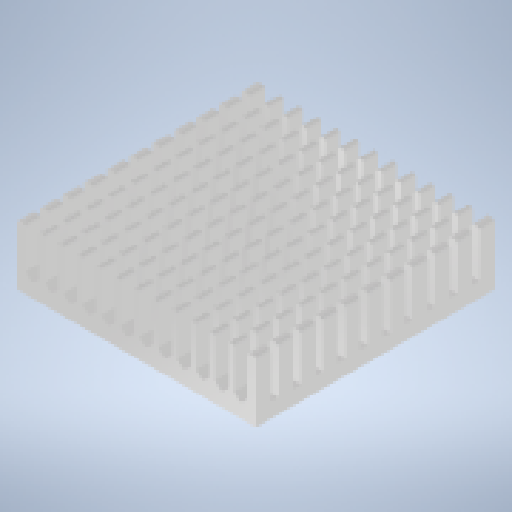
# Autodesk Inventor part: Nema17_CoolingElement
Saved by Autodesk Inventor 2023.1 (Build 271208000, 208)
## iProperties
Created: 2022-09-11
Part Number: Nema17_CoolingElement
Material: Generisch
Document SubType Name: Modeling
Designer: Rama
Density: 1 g/cm^3
Appearance: Aluminium - dunkel
Author: Rama
Autodesk Inventor part; units mm, degrees
ref_plane "YZ Plane" through (0, 0, 0) normal (1, 0, 0) x (0, 1, 0)
ref_plane "XZ Plane" through (0, 0, 0) normal (0, 1, 0) x (-1, 0, 0)
ref_plane "XY Plane" through (0, 0, 0) normal (0, 0, 1) x (1, 0, 0)
sketch "Skizze1" plane through (0, 0, 0) normal (0, 0, 1) x (1, 0, 0)
  line L0 (0, 4.4) -> (2, 4.4) projected
  line L1 (0, 0.4) -> (0, 4.4) projected
  line L2 (40.4, 0.4) -> (0, 0.4) projected
  line L3 (40.4, 0.4) -> (40.4, 4.4) projected
  line L4 (38.4, 4.4) -> (40.4, 4.4) projected
  line L5 (38.4, 3) -> (38.4, 4.4) projected
  line L6 (38, 2.6) -> (38.4, 3) projected
  line L7 (37.6, 2.6) -> (38, 2.6) projected
  line L8 (37.2, 3) -> (37.6, 2.6) projected
  line L9 (37.2, 3) -> (37.2, 4.4) projected
  line L10 (35.2, 4.4) -> (37.2, 4.4) projected
  line L11 (35.2, 3) -> (35.2, 4.4) projected
  line L12 (34.8, 2.6) -> (35.2, 3) projected
  line L13 (34.4, 2.6) -> (34.8, 2.6) projected
  line L14 (34, 3) -> (34.4, 2.6) projected
  line L15 (34, 3) -> (34, 4.4) projected
  line L16 (32, 4.4) -> (34, 4.4) projected
  line L17 (32, 3) -> (32, 4.4) projected
  line L18 (31.6, 2.6) -> (32, 3) projected
  line L19 (31.2, 2.6) -> (31.6, 2.6) projected
  line L20 (30.8, 3) -> (31.2, 2.6) projected
  line L21 (30.8, 3) -> (30.8, 4.4) projected
  line L22 (28.8, 4.4) -> (30.8, 4.4) projected
  line L23 (28.8, 3) -> (28.8, 4.4) projected
  line L24 (28.4, 2.6) -> (28.8, 3) projected
  line L25 (28, 2.6) -> (28.4, 2.6) projected
  line L26 (27.6, 3) -> (28, 2.6) projected
  line L27 (27.6, 3) -> (27.6, 4.4) projected
  line L28 (25.6, 4.4) -> (27.6, 4.4) projected
  line L29 (25.6, 3) -> (25.6, 4.4) projected
  line L30 (25.2, 2.6) -> (25.6, 3) projected
  line L31 (24.8, 2.6) -> (25.2, 2.6) projected
  line L32 (24.4, 3) -> (24.8, 2.6) projected
  line L33 (24.4, 3) -> (24.4, 4.4) projected
  line L34 (22.4, 4.4) -> (24.4, 4.4) projected
  line L35 (22.4, 3) -> (22.4, 4.4) projected
  line L36 (22, 2.6) -> (22.4, 3) projected
  line L37 (21.6, 2.6) -> (22, 2.6) projected
  line L38 (21.2, 3) -> (21.6, 2.6) projected
  line L39 (21.2, 3) -> (21.2, 4.4) projected
  line L40 (19.2, 4.4) -> (21.2, 4.4) projected
  line L41 (19.2, 3) -> (19.2, 4.4) projected
  line L42 (18.8, 2.6) -> (19.2, 3) projected
  line L43 (18.4, 2.6) -> (18.8, 2.6) projected
  line L44 (18, 3) -> (18.4, 2.6) projected
  line L45 (18, 3) -> (18, 4.4) projected
  line L46 (16, 4.4) -> (18, 4.4) projected
  line L47 (16, 3) -> (16, 4.4) projected
  line L48 (15.6, 2.6) -> (16, 3) projected
  line L49 (15.2, 2.6) -> (15.6, 2.6) projected
  line L50 (14.8, 3) -> (15.2, 2.6) projected
  line L51 (14.8, 3) -> (14.8, 4.4) projected
  line L52 (12.8, 4.4) -> (14.8, 4.4) projected
  line L53 (12.8, 3) -> (12.8, 4.4) projected
  line L54 (12.4, 2.6) -> (12.8, 3) projected
  line L55 (12, 2.6) -> (12.4, 2.6) projected
  line L56 (11.6, 3) -> (12, 2.6) projected
  line L57 (11.6, 3) -> (11.6, 4.4) projected
  line L58 (9.6, 4.4) -> (11.6, 4.4) projected
  line L59 (9.6, 3) -> (9.6, 4.4) projected
  line L60 (9.2, 2.6) -> (9.6, 3) projected
  line L61 (8.8, 2.6) -> (9.2, 2.6) projected
  line L62 (8.4, 3) -> (8.8, 2.6) projected
  line L63 (8.4, 3) -> (8.4, 4.4) projected
  line L64 (6.4, 4.4) -> (8.4, 4.4) projected
  line L65 (6.4, 3) -> (6.4, 4.4) projected
  line L66 (6, 2.6) -> (6.4, 3) projected
  line L67 (5.6, 2.6) -> (6, 2.6) projected
  line L68 (5.2, 3) -> (5.6, 2.6) projected
  line L69 (5.2, 3) -> (5.2, 4.4) projected
  line L70 (3.2, 4.4) -> (5.2, 4.4) projected
  line L71 (3.2, 3) -> (3.2, 4.4) projected
  line L72 (2.8, 2.6) -> (3.2, 3) projected
  line L73 (2.4, 2.6) -> (2.8, 2.6) projected
  line L74 (2, 3) -> (2.4, 2.6) projected
  line L75 (2, 3) -> (2, 4.4) projected
  line L76 (40.4, 0.4) -> (0, 0.4)
  line L77 (0, 0.4) -> (0, -0.4)
  line L78 (0, -0.4) -> (40.4, -0.4)
  line L79 (40.4, -0.4) -> (40.4, 0.4)
  point P0 (0, 0)
  dimension "d0" = 0.8
  constraints: 8 end point, 2 parallel, 1 horizontal, 1 perpendicular, 1 point on line
  measures "d0" distance between parallel lines of L76 L78
ref_plane "Arbeitsebene1" through (0, 0.4, 40.4) normal (0, 0, -1) x (0, 1, 0)
extrude "Extrusion1" add sketch "Skizze1" along normal up to surface (40.4 mm away)
chamfer "Fase1" distance 0.5 angle 45 4 edges at (0, -0.4, 20.2) (20.2, -0.4, 0) (40.4, -0.4, 20.2) (20.2, -0.4, 40.4)
move faces "Verschieben1" translate (0, 6, 0) faces at (1.3333, 4.4, 13.4667) (4.5333, 4.4, 13.4667) (7.7333, 4.4, 13.4667) (10.9333, 4.4, 13.4667) (14.1333, 4.4, 13.4667) (17.3333, 4.4, 13.4667) (20.5333, 4.4, 13.4667) (23.7333, 4.4, 13.4667) (26.9333, 4.4, 13.4667) (30.1333, 4.4, 13.4667) (33.3333, 4.4, 13.4667) (36.5333, 4.4, 13.4667) (39.7333, 4.4, 13.4667)
move faces "Verschieben2" translate (-0.5, 0, 0) faces at (37.2, 5.4667, 13.4667) (34, 5.4667, 13.4667) (30.8, 5.4667, 13.4667) (27.6, 5.4667, 13.4667) (24.4, 5.4667, 13.4667) (21.2, 5.4667, 13.4667) (18, 5.4667, 13.4667) (14.8, 5.4667, 13.4667) (11.6, 5.4667, 13.4667) (8.4, 5.4667, 13.4667) (5.2, 5.4667, 13.4667) (2, 5.4667, 13.4667)
move faces "Verschieben3" translate (0.5, 0, 0) faces at (3.2, 7.9333, 13.4667) (6.4, 7.9333, 13.4667) (9.6, 7.9333, 13.4667) (12.8, 5.4667, 26.9333) (16, 7.9333, 13.4667) (19.2, 5.4667, 26.9333) (22.4, 5.4667, 26.9333) (25.6, 7.9333, 13.4667) (28.8, 7.9333, 13.4667) (32, 7.9333, 13.4667) (35.2, 7.9333, 13.4667) (38.4, 7.9333, 13.4667)
fillet "Rundung1" radius 0.5 26 edges at (0, 10.4, 20.2) (1.5, 10.4, 20.2) (3.7, 10.4, 20.2) (4.7, 10.4, 20.2) (6.9, 10.4, 20.2) (7.9, 10.4, 20.2) (10.1, 10.4, 20.2) (11.1, 10.4, 20.2) (13.3, 10.4, 20.2) (14.3, 10.4, 20.2) (16.5, 10.4, 20.2) (17.5, 10.4, 20.2) (19.7, 10.4, 20.2) (20.7, 10.4, 20.2) (22.9, 10.4, 20.2) (23.9, 10.4, 20.2) (26.1, 10.4, 20.2) (27.1, 10.4, 20.2) (29.3, 10.4, 20.2) (30.3, 10.4, 20.2) (32.5, 10.4, 20.2) (33.5, 10.4, 20.2) (35.7, 10.4, 20.2) (36.7, 10.4, 20.2) (38.9, 10.4, 20.2) (40.4, 10.4, 20.2)
sketch "Skizze2" plane through (0, 0.1, 0) normal (-1, 0, 0) x (0, 0, 1)
  line L0 (0, 9.8) -> (40.4, 9.8) projected
  line L1 (0, 9.8) -> (0, 0) projected
  line L2 (40.4, 0) -> (0, 0) projected
  line L3 (40.4, 9.8) -> (40.4, 0) projected
  line L4 (37.9, 2.5) -> (36.61, 2.5)
  line L5 (36.61, 2.5) -> (36.61, 12.7645)
  line L6 (36.61, 12.7645) -> (37.9, 12.7645)
  line L7 (37.9, 12.7645) -> (37.9, 2.5)
  line L8 (34.11, 2.5) -> (32.82, 2.5)
  line L9 (32.82, 2.5) -> (32.82, 12.7645)
  line L10 (32.82, 12.7645) -> (34.11, 12.7645)
  line L11 (34.11, 12.7645) -> (34.11, 2.5)
  line L12 (30.32, 2.5) -> (29.03, 2.5)
  line L13 (29.03, 2.5) -> (29.03, 12.7645)
  line L14 (29.03, 12.7645) -> (30.32, 12.7645)
  line L15 (30.32, 12.7645) -> (30.32, 2.5)
  line L16 (26.53, 2.5) -> (25.24, 2.5)
  line L17 (25.24, 2.5) -> (25.24, 12.7645)
  line L18 (25.24, 12.7645) -> (26.53, 12.7645)
  line L19 (26.53, 12.7645) -> (26.53, 2.5)
  line L20 (22.74, 2.5) -> (21.45, 2.5)
  line L21 (21.45, 2.5) -> (21.45, 12.7645)
  line L22 (21.45, 12.7645) -> (22.74, 12.7645)
  line L23 (22.74, 12.7645) -> (22.74, 2.5)
  line L24 (18.95, 2.5) -> (17.66, 2.5)
  line L25 (17.66, 2.5) -> (17.66, 12.7645)
  line L26 (17.66, 12.7645) -> (18.95, 12.7645)
  line L27 (18.95, 12.7645) -> (18.95, 2.5)
  line L28 (15.16, 2.5) -> (13.87, 2.5)
  line L29 (13.87, 2.5) -> (13.87, 12.7645)
  line L30 (13.87, 12.7645) -> (15.16, 12.7645)
  line L31 (15.16, 12.7645) -> (15.16, 2.5)
  line L32 (11.37, 2.5) -> (10.08, 2.5)
  line L33 (10.08, 2.5) -> (10.08, 12.7645)
  line L34 (10.08, 12.7645) -> (11.37, 12.7645)
  line L35 (11.37, 12.7645) -> (11.37, 2.5)
  line L36 (7.58, 2.5) -> (6.29, 2.5)
  line L37 (6.29, 2.5) -> (6.29, 12.7645)
  line L38 (6.29, 12.7645) -> (7.58, 12.7645)
  line L39 (7.58, 12.7645) -> (7.58, 2.5)
  line L40 (3.79, 2.5) -> (2.5, 2.5)
  line L41 (2.5, 2.5) -> (2.5, 12.7645)
  line L42 (2.5, 12.7645) -> (3.79, 12.7645)
  line L43 (3.79, 12.7645) -> (3.79, 2.5)
  line L44 (0, 2.5) -> (40.4, 2.5) projected
  line L45 (0, 2.5) -> (40.4, 2.5) projected
  point P0 (0, -0.1)
  point P1 (37.255, 2.5)
  point P2 (33.465, 2.5)
  point P3 (29.675, 2.5)
  point P4 (25.885, 2.5)
  point P5 (22.095, 2.5)
  point P6 (18.305, 2.5)
  point P7 (14.515, 2.5)
  point P8 (10.725, 2.5)
  point P9 (6.935, 2.5)
  point P10 (3.145, 2.5)
  point P11 (37.255, 12.7645)
  point P12 (33.465, 12.7645)
  point P13 (29.675, 12.7645)
  point P14 (25.885, 12.7645)
  point P15 (22.095, 12.7645)
  point P16 (18.305, 12.7645)
  point P17 (14.515, 12.7645)
  point P18 (10.725, 12.7645)
  point P19 (6.935, 12.7645)
  dimension "d16" = 2.5
  dimension "d17" = 2.5
  dimension "d18" = 2.5
  dimension "d19" = 2.5
  dimension "d20" = 2.5
  dimension "d21" = 2.5
  dimension "d22" = 2.5
  dimension "d23" = 2.5
  dimension "d24" = 2.5
  dimension "d25" = 2.5
  dimension "d26" = 2.5
  dimension "d27" = 1.29
  dimension "d28" = 1.29
  dimension "d29" = 1.29
  dimension "d30" = 1.29
  dimension "d31" = 1.29
  dimension "d32" = 1.29
  dimension "d33" = 1.29
  dimension "d34" = 1.29
  dimension "d35" = 1.29
  dimension "d36" = 1.29
  constraints: 80 end point, 20 parallel, 19 midpoint, 19 point on line, 10 horizontal, 10 perpendicular
  measures "d16" distance between parallel lines of L3 L7
  measures "d17" distance between parallel lines of L11 L5
  measures "d18" distance between parallel lines of L15 L9
  measures "d19" distance between parallel lines of L19 L13
  measures "d20" distance between parallel lines of L23 L17
  measures "d21" distance between parallel lines of L27 L21
  measures "d22" distance between parallel lines of L31 L25
  measures "d23" distance between parallel lines of L35 L29
  measures "d24" distance between parallel lines of L39 L33
  measures "d25" distance between parallel lines of L43 L37
  measures "d26" distance between parallel lines of L1 L41
  measures "d27" distance of L5.end L6.end
  measures "d28" distance of L9.end L10.end
  measures "d29" distance of L41.end L42.end
  measures "d30" distance of L37.end L38.end
  measures "d31" distance of L33.end L34.end
  measures "d32" distance of L29.end L30.end
  measures "d33" distance of L25.end L26.end
  measures "d34" distance of L21.end L22.end
  measures "d35" distance of L17.end L18.end
  measures "d36" distance of L13.end L14.end
extrude "Extrusion2" cut sketch "Skizze2" against normal through all contours L41 L42 L43 L0 | L0 L43 L40 L41 | L37 L38 L39 L0 | L0 L39 L36 L37 | L33 L34 L35 L0 | L0 L35 L32 L33 | L4 L5 L0 L7 | L0 L5 L6 L7 | L29 L30 L31 L0 | L0 L31 L28 L29 | L8 L9 L0 L11 | L0 L9 L10 L11 | L25 L26 L27 L0 | L0 L27 L24 L25 | L12 L13 L0 L15 | L0 L13 L14 L15 | L21 L22 L23 L0 | L0 L23 L20 L21 | L16 L17 L0 L19 | L0 L17 L18 L19
equation "\"d17\" = d16"
equation "\"d18\" = d16"
equation "\"d19\" = d16"
equation "\"d20\" = d16"
equation "\"d21\" = d16"
equation "\"d22\" = d16"
equation "\"d23\" = d16"
equation "\"d24\" = d16"
equation "\"d25\" = d16"
equation "\"d26\" = d16"
equation "\"d27\" = d36"
equation "\"d28\" = d27"
equation "\"d29\" = d27"
equation "\"d30\" = d27"
equation "\"d31\" = d27"
equation "\"d32\" = d27"
equation "\"d33\" = d27"
equation "\"d34\" = d27"
equation "\"d35\" = d27"
